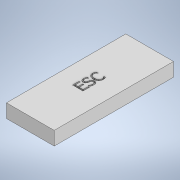
# Autodesk Inventor part: ESC
Saved by Autodesk Inventor 2022.1 (Build 261234020, 234B)
## iProperties
Created: 2021-11-21
Part Number: ESC
Material: Generic
Document SubType Name: Modeling
Designer: Alexander
Density: 1 g/cm^3
Appearance: Default
Author: Alexander
Autodesk Inventor part; units mm, degrees
note: some values were not read from the file. Chosen so that the rebuilt part matches the saved one: direction of "Emboss1".
ref_plane "YZ Plane" through (0, 0, 0) normal (1, 0, 0) x (0, 1, 0)
ref_plane "XZ Plane" through (0, 0, 0) normal (0, 1, 0) x (-1, 0, 0)
ref_plane "XY Plane" through (0, 0, 0) normal (0, 0, 1) x (1, 0, 0)
sketch "Sketch1" plane through (0, 0, 0) normal (0, 1, 0) x (-1, 0, 0)
  line L0 (-14, -35) -> (14, -35)
  line L1 (14, -35) -> (14, 35)
  line L2 (14, 35) -> (-14, 35)
  line L3 (-14, 35) -> (-14, -35)
  line L4 (-14, -35) -> (14, 35) construction
  line L5 (14, -35) -> (-14, 35) construction
  point P0 (0, 0)
  dimension "d0" = 28
  dimension "d1" = 70
  constraints: 12 end point, 2 midpoint, 2 parallel, 1 horizontal, 1 perpendicular
  measures "d0" distance of L2.end L1.end
  measures "d1" distance of L1.end L0.end
extrude "Extrusion1" add sketch "Sketch1" along normal blind 8
sketch "Sketch2" plane through (0, 8, 0) normal (0, 1, 0) x (1, 0, 0)
  line L0 (-3.7383, -7.2249) -> (-3.7383, 52.4053) construction
  line L1 (-3.7383, 52.4053) -> (19.2336, 52.4053) construction
  line L2 (19.2336, 52.4053) -> (19.2336, -7.2249) construction
  line L3 (19.2336, -7.2249) -> (-3.7383, -7.2249) construction
  line L4 (2.4705, -6.607) -> (-3.6295, -6.607)
  line L5 (-3.6295, -6.607) -> (-3.6295, -2.7908)
  line L6 (-3.6295, -2.7908) -> (-2.9078, -2.7908)
  line L7 (-2.9078, -2.7908) -> (-2.9078, -5.7963)
  line L8 (-2.9078, -5.7963) -> (-1.237, -5.7963)
  line L9 (-1.237, -5.7963) -> (-1.237, -2.9935)
  line L10 (-1.237, -2.9935) -> (-0.5152, -2.9935)
  line L11 (-0.5152, -2.9935) -> (-0.5152, -5.7963)
  line L12 (-0.5152, -5.7963) -> (1.7488, -5.7963)
  line L13 (1.7488, -5.7963) -> (1.7488, -2.7908)
  line L14 (1.7488, -2.7908) -> (2.4705, -2.7908)
  line L15 (2.4705, -2.7908) -> (2.4705, -6.607)
  spline S0 degree 2 poles (2.5792, -0.2005) (2.5792, -0.8629) (2.3024, -1.7922) (2.1047, -2.2025) knots 0 0 0 1 2 2 2
  line L16 (2.1047, -2.2025) -> (1.0864, -2.2025)
  line L17 (1.0864, -2.2025) -> (1.0864, -2.1432)
  spline S1 degree 2 poles (1.0864, -2.1432) (1.4621, -1.7428) (1.8773, -0.7294) (1.8773, -0.2598) knots 0 0 0 1 2 2 2
  spline S2 degree 2 poles (1.8773, -0.2598) (1.8773, 0.4125) (1.3187, 1.0996) (0.859, 1.0996) knots 0 0 0 1 2 2 2
  spline S3 degree 2 poles (0.859, 1.0996) (0.4932, 1.0996) (0.0384, 0.7387) (-0.0753, 0.3482) knots 0 0 0 1 2 2 2
  spline S4 degree 2 poles (-0.0753, 0.3482) (-0.1544, 0.0664) (-0.2631, -0.4032) (-0.3521, -0.7541) knots 0 0 0 1 2 2 2
  spline S5 degree 2 poles (-0.3521, -0.7541) (-0.4362, -1.0705) (-0.6883, -1.5698) (-0.8909, -1.7626) knots 0 0 0 1 2 2 2
  spline S6 degree 2 poles (-0.8909, -1.7626) (-1.0936, -1.9504) (-1.6374, -2.158) (-1.9933, -2.158) knots 0 0 0 1 2 2 2
  spline S7 degree 2 poles (-1.9933, -2.158) (-2.7348, -2.158) (-3.7383, -1.0013) (-3.7383, -0.1066) knots 0 0 0 1 2 2 2
  spline S8 degree 2 poles (-3.7383, -0.1066) (-3.7383, 0.4075) (-3.5356, 1.3171) (-3.3428, 1.7076) knots 0 0 0 1 2 2 2
  line L18 (-3.3428, 1.7076) -> (-2.3739, 1.7076)
  line L19 (-2.3739, 1.7076) -> (-2.3739, 1.6483)
  spline S9 degree 2 poles (-2.3739, 1.6483) (-2.6409, 1.3566) (-3.0363, 0.4471) (-3.0363, -0.0522) knots 0 0 0 1 2 2 2
  spline S10 degree 2 poles (-3.0363, -0.0522) (-3.0363, -0.6157) (-2.5074, -1.3127) (-2.0773, -1.3127) knots 0 0 0 1 2 2 2
  spline S11 degree 2 poles (-2.0773, -1.3127) (-1.6917, -1.3127) (-1.232, -0.9024) (-1.1282, -0.5169) knots 0 0 0 1 2 2 2
  spline S12 degree 2 poles (-1.1282, -0.5169) (-1.059, -0.2598) (-0.881, 0.4866) (-0.8069, 0.7338) knots 0 0 0 1 2 2 2
  spline S13 degree 2 poles (-0.8069, 0.7338) (-0.6141, 1.3616) (0.162, 1.9449) (0.7305, 1.9449) knots 0 0 0 1 2 2 2
  spline S14 degree 2 poles (0.7305, 1.9449) (1.0913, 1.9449) (1.7834, 1.6532) (2.0256, 1.3912) knots 0 0 0 1 2 2 2
  spline S15 degree 2 poles (2.0256, 1.3912) (2.2925, 1.0996) (2.5792, 0.3581) (2.5792, -0.2005) knots 0 0 0 1 2 2 2
  spline S16 degree 2 poles (2.5792, 5.1531) (2.5792, 4.5599) (2.1788, 3.5564) (1.7784, 3.1906) knots 0 0 0 1 2 2 2
  spline S17 degree 2 poles (1.7784, 3.1906) (1.383, 2.8248) (0.1966, 2.4244) (-0.5746, 2.4244) knots 0 0 0 1 2 2 2
  spline S18 degree 2 poles (-0.5746, 2.4244) (-1.3408, 2.4244) (-2.4777, 2.8149) (-2.8979, 3.1856) knots 0 0 0 1 2 2 2
  spline S19 degree 2 poles (-2.8979, 3.1856) (-3.3082, 3.5514) (-3.7383, 4.55) (-3.7383, 5.1679) knots 0 0 0 1 2 2 2
  spline S20 degree 2 poles (-3.7383, 5.1679) (-3.7383, 5.4744) (-3.6493, 6.0132) (-3.5801, 6.2406) knots 0 0 0 1 2 2 2
  spline S21 degree 2 poles (-3.5801, 6.2406) (-3.5158, 6.4383) (-3.3329, 6.8486) (-3.2242, 7.0513) knots 0 0 0 1 2 2 2
  line L20 (-3.2242, 7.0513) -> (-2.2454, 7.0513)
  line L21 (-2.2454, 7.0513) -> (-2.2454, 6.987)
  spline S22 degree 2 poles (-2.2454, 6.987) (-2.3443, 6.8783) (-2.6211, 6.5421) (-2.7545, 6.2999) knots 0 0 0 1 2 2 2
  spline S23 degree 2 poles (-2.7545, 6.2999) (-2.8831, 6.0676) (-3.0462, 5.5189) (-3.0462, 5.163) knots 0 0 0 1 2 2 2
  spline S24 degree 2 poles (-3.0462, 5.163) (-3.0462, 4.7724) (-2.7249, 4.0754) (-2.4184, 3.8134) knots 0 0 0 1 2 2 2
  spline S25 degree 2 poles (-2.4184, 3.8134) (-2.107, 3.5564) (-1.1628, 3.2697) (-0.5746, 3.2697) knots 0 0 0 1 2 2 2
  spline S26 degree 2 poles (-0.5746, 3.2697) (0.0532, 3.2697) (0.9579, 3.5712) (1.2693, 3.8332) knots 0 0 0 1 2 2 2
  spline S27 degree 2 poles (1.2693, 3.8332) (1.5708, 4.0903) (1.8773, 4.7774) (1.8773, 5.163) knots 0 0 0 1 2 2 2
  spline S28 degree 2 poles (1.8773, 5.163) (1.8773, 5.5139) (1.7043, 6.1121) (1.5758, 6.3444) knots 0 0 0 1 2 2 2
  spline S29 degree 2 poles (1.5758, 6.3444) (1.4472, 6.5668) (1.1803, 6.898) (1.0864, 6.992) knots 0 0 0 1 2 2 2
  line L22 (1.0864, 6.992) -> (1.0864, 7.0513)
  line L23 (1.0864, 7.0513) -> (2.0553, 7.0513)
  spline S30 degree 2 poles (2.0553, 7.0513) (2.1492, 6.8486) (2.3222, 6.4927) (2.4013, 6.2406) knots 0 0 0 1 2 2 2
  spline S31 degree 2 poles (2.4013, 6.2406) (2.4903, 5.9736) (2.5792, 5.5189) (2.5792, 5.1531) knots 0 0 0 1 2 2 2
  point P0 (0, 0)
  constraints: 2 other
emboss "Emboss1" sketch "Sketch2" operation cut depth 1 direction (0, -1, 0)
body "Solid1"
